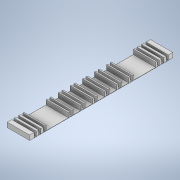
# Autodesk Inventor part: wire_holder_middle
Saved by Autodesk Inventor 2021 (Build 250183000, 183)
## iProperties
Created: 2021-02-03
Part Number: wire_holder_middle
Material: Generic
Document SubType Name: Modeling
Designer: User
Density: 1 g/cm^3
Appearance: Default
Author: User
Autodesk Inventor part; units mm, degrees
ref_plane "YZ Plane" through (0, 0, 0) normal (1, 0, 0) x (0, 1, 0)
ref_plane "XZ Plane" through (0, 0, 0) normal (0, 1, 0) x (-1, 0, 0)
ref_plane "XY Plane" through (0, 0, 0) normal (0, 0, 1) x (1, 0, 0)
sketch "Sketch1" plane through (0, 0, 0) normal (0, 1, 0) x (-1, 0, 0)
  line L0 (49.0311, 150) -> (99.0311, 150)
  line L1 (49.0311, 145) -> (99.0311, 145)
  line L2 (99.0311, 16) -> (49.0311, 16)
  line L3 (99.0311, 11) -> (49.0311, 11)
  line L4 (49.0311, 135) -> (99.0311, 135)
  line L5 (49.0311, 140) -> (99.0311, 140)
  line L6 (99.0311, 43) -> (49.0311, 43)
  line L7 (99.0311, 38) -> (49.0311, 38)
  line L8 (49.0311, 125) -> (99.0311, 125)
  line L9 (99.0311, 70) -> (49.0311, 70)
  line L10 (49.0311, 130) -> (99.0311, 130)
  line L11 (99.0311, 65) -> (49.0311, 65)
  line L12 (49.0311, -11) -> (99.0311, -11)
  line L13 (99.0311, -150) -> (49.0311, -150)
  line L14 (49.0311, -16) -> (99.0311, -16)
  line L15 (99.0311, -145) -> (49.0311, -145)
  line L16 (49.0311, -38) -> (99.0311, -38)
  line L17 (99.0311, -140) -> (49.0311, -140)
  line L18 (49.0311, -43) -> (99.0311, -43)
  line L19 (99.0311, -135) -> (49.0311, -135)
  line L20 (49.0311, -65) -> (99.0311, -65)
  line L21 (49.0311, -70) -> (99.0311, -70)
  line L22 (99.0311, -125) -> (49.0311, -125)
  line L23 (99.0311, -130) -> (49.0311, -130)
  line L24 (99.0311, -160) -> (49.0311, -160)
  line L25 (49.0311, 160) -> (99.0311, 160)
  line L26 (99.0311, -231.4683) -> (49.0311, -231.4683) construction
  line L27 (49.0311, -231.4683) -> (49.0311, 236.8413) construction
  line L28 (49.0311, 236.8413) -> (99.0311, 236.8413) construction
  line L29 (99.0311, 236.8413) -> (99.0311, -231.4683) construction
  line L30 (99.0311, -160) -> (49.0311, -160)
  line L31 (49.0311, -160) -> (49.0311, 160)
  line L32 (49.0311, 160) -> (99.0311, 160)
  line L33 (99.0311, 160) -> (99.0311, -160)
  point P0 (-18.4221, 150)
  dimension "d3" = 5
  dimension "d5" = 5
  dimension "d7" = 5
  dimension "d9" = 5
  dimension "d14" = 5
  dimension "d16" = 5
  dimension "d18" = 5
  dimension "d20" = 22
  dimension "d22" = 5
  dimension "d30" = 5
  dimension "d32" = 5
  dimension "d38" = 5
  dimension "d40" = 5
  dimension "d43" = 5
  dimension "d48" = 5
  dimension "d49" = 5
  dimension "d56" = 10
  dimension "d58" = 10
  dimension "d63" = 50
  constraints: 60 end point, 13 horizontal, 7 parallel, 64 other
  measures "d3" distance between parallel lines of L0 L1
  measures "d5" distance between parallel lines of L5 L1
  measures "d7" distance between parallel lines of L3 L2
  measures "d9" distance between parallel lines of L5 L4
  measures "d14" distance between parallel lines of L7 L6
  measures "d16" distance between parallel lines of L4 L10
  measures "d18" distance between parallel lines of L10 L8
  measures "d20" distance between parallel lines of L6 L11
  measures "d22" distance between parallel lines of L11 L9
  measures "d30" distance between parallel lines of L14 L12
  measures "d32" distance between parallel lines of L13 L15
  measures "d38" distance between parallel lines of L16 L18
  measures "d40" distance between parallel lines of L17 L19
  measures "d43" distance between parallel lines of L20 L21
  measures "d48" distance between parallel lines of L23 L22
  measures "d49" distance between parallel lines of L19 L23
  measures "d56" distance between parallel lines of L24 L13
  measures "d58" distance between parallel lines of L0 L25
  measures "d63" distance of L28.start L28.end
extrude "Extrusion1" add sketch "Sketch1" along normal blind 10 contours L31 L25 L33 L0 | L1 L33 L5 L31 | L4 L33 L10 L31 | L8 L33 L9 L31 | L11 L33 L6 L31 | L7 L33 L2 L31 | L3 L33 L12 L31 | L14 L33 L16 L31 | L18 L33 L20 L31 | L21 L33 L22 L31 | L23 L33 L19 L31 | L17 L33 L15 L31 | L13 L33 L24 L31
sketch "Sketch2" plane through (0, 10, 0) normal (0, 1, 0) x (1, 0, 0)
  line L0 (-99.0311, 125) -> (-99.0311, 70) projected
  line L1 (-49.0311, 70) -> (-49.0311, 125) projected
  line L2 (-99.0311, 122) -> (-49.0311, 122)
  line L3 (-49.0311, 122) -> (-49.0311, 73)
  line L4 (-49.0311, 73) -> (-99.0311, 73)
  line L5 (-99.0311, 73) -> (-99.0311, 122)
  line L6 (-49.0311, 125) -> (-99.0311, 125) projected
  line L7 (-99.0311, 70) -> (-49.0311, 70) projected
  line L8 (-99.0311, 65) -> (-99.0311, 43) projected
  line L9 (-99.0311, 62) -> (-49.0311, 62)
  line L10 (-49.0311, 62) -> (-49.0311, 46)
  line L11 (-49.0311, 46) -> (-99.0311, 46)
  line L12 (-99.0311, 46) -> (-99.0311, 62)
  line L13 (-99.0311, 35) -> (-49.0311, 35)
  line L14 (-49.0311, 35) -> (-49.0311, 19)
  line L15 (-49.0311, 19) -> (-99.0311, 19)
  line L16 (-99.0311, 19) -> (-99.0311, 35)
  line L17 (-49.0311, -11) -> (-49.0311, 11) projected
  line L18 (-99.0311, 8) -> (-49.0311, 8)
  line L19 (-49.0311, 8) -> (-49.0311, -8)
  line L20 (-49.0311, -8) -> (-99.0311, -8)
  line L21 (-99.0311, -8) -> (-99.0311, 8)
  line L22 (-99.0311, -19) -> (-49.0311, -19)
  line L23 (-49.0311, -19) -> (-49.0311, -35)
  line L24 (-49.0311, -35) -> (-99.0311, -35)
  line L25 (-99.0311, -35) -> (-99.0311, -19)
  line L26 (-99.0311, -43) -> (-99.0311, -65) projected
  line L27 (-49.0311, -65) -> (-49.0311, -43) projected
  line L28 (-99.0311, -46) -> (-49.0311, -46)
  line L29 (-49.0311, -46) -> (-49.0311, -62)
  line L30 (-49.0311, -62) -> (-99.0311, -62)
  line L31 (-99.0311, -62) -> (-99.0311, -46)
  line L32 (-49.0311, -125) -> (-49.0311, -70) projected
  line L33 (-99.0311, -73) -> (-49.0311, -73)
  line L34 (-49.0311, -73) -> (-49.0311, -122)
  line L35 (-49.0311, -122) -> (-99.0311, -122)
  line L36 (-99.0311, -122) -> (-99.0311, -73)
  line L37 (-49.0311, 65) -> (-99.0311, 65) projected
  line L38 (-99.0311, 43) -> (-49.0311, 43) projected
  line L39 (-49.0311, 38) -> (-99.0311, 38) projected
  line L40 (-99.0311, 16) -> (-49.0311, 16) projected
  line L41 (-49.0311, 11) -> (-99.0311, 11) projected
  line L42 (-99.0311, -11) -> (-49.0311, -11) projected
  line L43 (-49.0311, -16) -> (-99.0311, -16) projected
  line L44 (-99.0311, -38) -> (-49.0311, -38) projected
  line L45 (-49.0311, -43) -> (-99.0311, -43) projected
  line L46 (-99.0311, -65) -> (-49.0311, -65) projected
  line L47 (-49.0311, -70) -> (-99.0311, -70) projected
  line L48 (-99.0311, -125) -> (-49.0311, -125) projected
  point P0 (0, 0)
  dimension "d66" = 3
  dimension "d67" = 3
  dimension "d68" = 3
  dimension "d69" = 3
  dimension "d70" = 3
  dimension "d71" = 3
  dimension "d72" = 3
  dimension "d73" = 3
  dimension "d74" = 3
  dimension "d75" = 3
  dimension "d76" = 3
  dimension "d77" = 3
  dimension "d78" = 3
  dimension "d79" = 3
  constraints: 56 end point, 14 parallel, 13 point on line, 7 horizontal, 7 perpendicular
  measures "d66" distance between parallel lines of L6 L2
  measures "d67" distance between parallel lines of L7 L4
  measures "d68" distance between parallel lines of L9 L37
  measures "d69" distance between parallel lines of L38 L11
  measures "d70" distance between parallel lines of L13 L39
  measures "d71" distance between parallel lines of L40 L15
  measures "d72" distance between parallel lines of L18 L41
  measures "d73" distance between parallel lines of L42 L20
  measures "d74" distance between parallel lines of L22 L43
  measures "d75" distance between parallel lines of L44 L24
  measures "d76" distance between parallel lines of L28 L45
  measures "d77" distance between parallel lines of L46 L30
  measures "d78" distance between parallel lines of L33 L47
  measures "d79" distance between parallel lines of L48 L35
extrude "Extrusion2" cut sketch "Sketch2" against normal blind 10 contours L2 L1 L4 L0 | L9 L10 L11 L8 | L13 L14 L15 L16 | L20 L21 L18 L17 | L22 L23 L24 L25 | L28 L27 L30 L26 | L35 L36 L33 L32
sketch "Sketch3" plane through (-49.0311, 0, -150) normal (1, 0, 0) x (0, 0, -1)
  line L0 (10, 0) -> (10, 10) projected
  line L1 (10, 0) -> (-310, 0)
  line L2 (-310, 0) -> (-310, -0.5)
  line L3 (-310, -0.5) -> (10, -0.5)
  line L4 (10, -0.5) -> (10, 0)
  point P0 (-150, 0)
  dimension "d82" = 0.5
  constraints: 8 end point, 2 parallel, 1 horizontal, 1 perpendicular
  measures "d82" distance of L1.end L2.end
extrude "Extrusion3" add sketch "Sketch3" against normal blind 50
equation "\"d3\" = d25"
equation "\"d5\" = d26"
equation "\"d7\" = d25"
equation "\"d9\" = d25"
equation "\"d14\" = d25"
equation "\"d16\" = d26"
equation "\"d18\" = d25"
equation "\"d20\" = d28"
equation "\"d22\" = d25"
equation "\"d30\" = d51"
equation "\"d32\" = d51"
equation "\"d38\" = d51"
equation "\"d40\" = d51"
equation "\"d43\" = d51"
equation "\"d48\" = d51"
equation "\"d49\" = d53"
equation "\"d25\" = 5"
equation "\"d26\" = 5"
equation "\"d28\" = -1.2 * d25 + 0.2 * d29"
equation "\"d51\" = 5"
equation "\"d53\" = 5"
equation "\"d54\" = -1.2 * d51 + 0.2 * d55"
equation "\"d29\" = 140"
equation "\"d55\" = 140"
body "Solid1"
